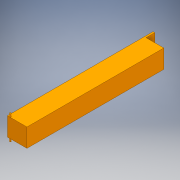
# Autodesk Inventor part: Batt_pillar
Saved by Autodesk Inventor 2018 (Build 220112000, 112)
## iProperties
Created: 2018-05-25
Part Number: Batt_pillar
Material: Generic
Document SubType Name: Modeling
Designer: Suchanek
Density: 1 g/cm^3
Appearance: Default
Author: Suchanek
Autodesk Inventor part; units mm, degrees
ref_plane "YZ Plane" through (0, 0, 0) normal (1, 0, 0) x (0, 1, 0)
ref_plane "XZ Plane" through (0, 0, 0) normal (0, 1, 0) x (-1, 0, 0)
ref_plane "XY Plane" through (0, 0, 0) normal (0, 0, 1) x (1, 0, 0)
sketch "Sketch1" plane through (0, 0, 0) normal (0, 0, 1) x (1, 0, 0)
  line L0 (1.2, 100) -> (0, 100)
  line L1 (0, 100) -> (0, 0)
  line L2 (0, 0) -> (1.2, 0)
  line L3 (1.2, 0) -> (1.2, 100)
  line L4 (1.2, 0) -> (13.4, 0)
  line L5 (13.4, 0) -> (13.4, 94)
  line L6 (13.4, 94) -> (1.2, 94)
  line L7 (1.2, 94) -> (1.2, 0)
  dimension "d0" = 1.2
  dimension "d1" = 100
  dimension "d2" = 12.2
  dimension "d3" = 94
  constraints: 16 end point, 4 parallel, 2 horizontal, 2 perpendicular
  measures "d0" distance of L1.end L2.end
  measures "d1" distance of L0.end L1.end
  measures "d2" distance of L6.end L5.end
  measures "d3" distance of L5.end L4.end
extrude "Extrusion1" add sketch "Sketch1" along normal blind 12.7
sketch "Sketch2" plane through (0, 0, 12.7) normal (0, 0, 1) x (1, 0, 0)
  circle A0 centre (1.5, 0.5) radius 0.5
  line L0 (0, 0) -> (13.4, 0) projected
  line L1 (0, 100) -> (0, 0) projected
  dimension "d6" = 1
  dimension "d7" = 1.5
  constraints: 1 centre point, 1 tangent
  measures "d6" diameter of A0
  measures "d7" distance from line of L1 A0.centre
extrude "Extrusion2" add sketch "Sketch2" along normal blind 2 and the other way blind 14.7
body "Solid1"
